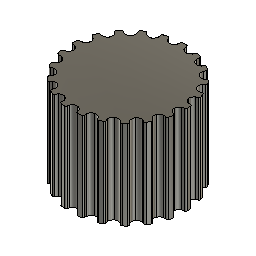
gear_21z (Autodesk Fusion 360 design; units mm, degrees)
Autodesk Fusion 360 part; units mm, degrees
sketch "Sketch1" plane through (0, 0, 0) normal (0, 0, 1) x (1, 0, 0) in component "gt2 pulley"
  circle A0 centre (0, 0) radius 6.6845 construction
  circle A1 centre (0, 0) radius 5.6805 construction
  line L0 (0, 0) -> (0, 6.6845) construction
  line L1 (0, 0) -> (0.9963, 6.6098) construction
  line L2 (0, 0) -> (1.4116, 6.5338) construction
  circle A2 centre (0, 0) radius 6.4305 construction
  arc A3 (0.358, 6.2782) -> (0.3948, 6.0167) centre (1.358, 6.2855) ccw
  circle A4 centre (0, 0) radius 6.2805 construction
  arc A5 (0.2129, 6.427) -> (0, 6.4305) centre (0, 0) ccw
  arc A6 (0.358, 6.2782) -> (0.2129, 6.427) centre (0.208, 6.2771) ccw
  arc A7 (0.3948, 6.0167) -> (0.8466, 5.6171) centre (0.9294, 6.1659) ccw
  arc A8 (0, 6.4305) -> (-0.2129, 6.427) centre (0, 0) ccw
  arc A9 (-0.2129, 6.427) -> (-0.358, 6.2782) centre (-0.208, 6.2771) ccw
  arc A10 (-0.3948, 6.0167) -> (-0.358, 6.2782) centre (-1.358, 6.2855) ccw
  arc A11 (-0.8464, 5.6171) -> (-0.3948, 6.0167) centre (-0.9294, 6.1659) ccw
  arc A12 (0.8466, 5.6171) -> (-0.8466, 5.6171) centre (0, 0) ccw
  point P0 (1.358, 6.2855)
  point P1 (0, 6.4305)
  dimension "d18" = 13.369
  dimension "d19" = 8.571
  dimension "d22" = 1.004
  dimension "d24" = 0.75
  dimension "d26" = 1
  dimension "d27" = 0.15
  dimension "d28" = 0.15
  dimension "d47" = 0.555
  dimension "d52" = 3.812
  constraint coincident A0.centre A1.centre
  constraint coincident A0 L0.end
  constraint vertical L0
  constraint coincident A0 L1.end
  constraint coincident A0 L2.end
  constraint concentric A1 A2
  constraint coincident A1 A7.end
  constraint coincident L1 A7.end
  constraint coincident A2 P0
  constraint coincident L2 P0
  constraint coincident P0 A3.centre
  constraint coincident A2 P1
  constraint coincident L0 P1
  constraint concentric A2 A4
  constraint coincident P1 A5.end
  constraint coincident A4 A6.centre
  constraint coincident A3.start A6.start
  constraint tangent A3 A6
  constraint tangent A3 A7
  constraint symmetric L0 A7.end A12.end
  constraint symmetric L0 A3.start A9.end
  constraint symmetric L0 A3.end A10.start
  constraint symmetric L0 A3 A10
  constraint symmetric L0 A5.start A8.end
  constraint symmetric L0 P1 A5.end
  constraint symmetric L0 A5 A8
  constraint symmetric L0 A6 A9
  constraint symmetric L0 A7 A11
  constraint coincident A1 A11.start
  constraint tangent A1 A7
  constraint coincident L1 A7.centre
  measures "d18" diameter of A0
  measures "d19" angle of L0 L1
  measures "d22" distance of A0 A1
  measures "d24" distance of A1 A2
  measures "d26" radius of A3
  measures "d27" distance of A2 A4
  measures "d28" radius of A6
  measures "d47" radius of A7
extrude "Extrude1" add sketch "Sketch1" along normal blind 10 makes body 1
pattern_circular "C-Pattern1" count 21 over 360 about axis through (0, 0, 1.75) along (0, 0, 1) of bodies 1 makes body 2 at (-2.293, 5.1971, 6.6667) makes body 3 at (-3.7231, 4.2903, 6.6667) makes body 4 at (-4.8222, 3.0023, 6.6667) makes body 5 at (-5.0973, 2.5072, 6.6667) makes body 6 at (-5.6756, -0.2358, 6.6667) makes body 7 at (-5.6474, -0.6125, 3.3333) makes body 8 at (-4.5566, -3.392, 6.6667) makes body 9 at (-3.7941, -4.2277, 6.6667) makes body 10 at (-3.0422, -4.7972, 3.3333) makes body 11 at (-0.7533, -5.6303, 6.6667) makes body 12 at (1.4928, -5.4808, 6.6667) makes body 13 at (1.8538, -5.3695, 3.3333) makes body 14 at (3.3542, -4.5845, 3.3333) makes body 15 at (4.5565, -3.3922, 3.3333) makes body 16 at (5.6474, -0.6127, 6.6667) makes body 17 at (5.6756, -0.236, 3.3333) makes body 18 at (5.0112, 2.675, 6.6667) makes body 19 at (4.0001, 4.0333, 6.6667) makes body 20 at (3.7232, 4.2902, 3.3333) makes body 21 at (2.2932, 5.197, 3.3333)
sketch "Sketch2" plane through (0, 0, 10) normal (0, 0, 1) x (-1, 0, 0)
  arc A0 (-3.8324, -4.9856) -> (-3.7964, -5.1903) centre (-3.7079, -5.0692) ccw
  arc A1 (-3.7964, -5.1903) -> (-3.4445, -5.4302) centre (0, 0) ccw
  arc A2 (-3.4445, -5.4302) -> (-3.2408, -5.3889) centre (-3.3641, -5.3035) ccw
  arc A3 (-3.0631, -5.1936) -> (-3.2408, -5.3889) centre (-2.4187, -5.9583) ccw
  arc A4 (-2.4649, -5.1179) -> (-3.0631, -5.1936) centre (-2.7055, -5.618) ccw
  arc A5 (-3.8637, -4.1641) -> (-2.4649, -5.1179) centre (0, 0) ccw
  arc A6 (-3.7155, -4.7488) -> (-3.8637, -4.1641) centre (-4.2412, -4.571) ccw
  arc A7 (-3.8324, -4.9856) -> (-3.7155, -4.7488) centre (-4.6628, -4.4283) ccw
  circle A8 centre (0, 0) radius 5.6805
  constraint concentric A1 A8
extrude "Extrude2" add sketch "Sketch2" against normal blind 10 contours A5 A8 bodies 1 2 3 4 5 6 7 8 9 10 11 12 13 14 15 16 17 18 19 20 21
extrude "Extrude4" [suppressed] in component "gt2 pulley"
pattern_circular "C-Pattern7" [suppressed] in component "gt2 pulley"
extrude "Extrude3" [suppressed] in component "gt2 pulley"
pattern_circular "C-Pattern6" [suppressed] in component "gt2 pulley"
extrude "Extrude2'" [suppressed] in component "gt2 pulley"
pattern_circular "C-Pattern5" [suppressed] in component "gt2 pulley"
extrude "Extrude1'" [suppressed] in component "gt2 pulley"
pattern_circular "C-Pattern4" [suppressed] in component "gt2 pulley"
pattern_circular "C-Pattern3" [suppressed] in component "gt2 pulley"
pattern_circular "C-Pattern2" [suppressed] in component "gt2 pulley"
pattern_circular "C-Pattern1'" [suppressed] in component "gt2 pulley"
copy_body "Body->Comp1" [suppressed] in component "Component"
copy_body "Body->Comp2" [suppressed] in component "Component'"
copy_body "Body->Comp3" [suppressed] in component "Component''"
copy_body "Body->Comp4" [suppressed] in component "Component'''"
copy_body "Body->Comp5" [suppressed] in component "Component''''"
copy_body "Body->Comp6" [suppressed] in component "Component'''''"
copy_body "Body->Comp7" [suppressed] in component "Component''''''"
copy_body "Body->Comp8" [suppressed] in component "Component'''''''"
copy_body "Body->Comp9" [suppressed] in component "Component''''''''"
copy_body "Body->Comp10" [suppressed] in component "Component'''''''''"
copy_body "Body->Comp11" [suppressed] in component "Component''''''''''"
copy_body "Body->Comp12" [suppressed] in component "Component'''''''''''"
copy_body "Body->Comp13" [suppressed] in component "Component''''''''''''"
copy_body "Body->Comp14" [suppressed] in component "Component'''''''''''''"
copy_body "Body->Comp15" [suppressed] in component "Component''''''''''''''"
copy_body "Body->Comp16" [suppressed] in component "Component'''''''''''''''"
copy_body "Body->Comp17" [suppressed] in component "Component''''''''''''''''"
copy_body "Body->Comp18" [suppressed] in component "Component'''''''''''''''''"
copy_body "Body->Comp19" [suppressed] in component "Component''''''''''''''''''"
copy_body "Body->Comp20" [suppressed] in component "Component'''''''''''''''''''"
component "gt2 pulley" placed x (1, 0, 0) y (0, 1, 0) z (0, 0, 1) at (0, 0, 0)
equation "NumTeeth = 21" comment "min 20"
equation "ToothPitch = 2 mm"
equation "PullyDia = NumTeeth * ToothPitch / PI"
equation "ToothAng = ( ( 360 / NumTeeth ) * 1 deg )"
equation "TransOffsetAngle = ToothAng * 0.2"
equation "Sholulder_Radius = 0.15 mm"
equation "Root_Radius = 0.555 mm"
equation "TransRadius = 1 mm"
equation "ToolHeight = 0.75 mm"
equation "PLD = 0.254 mm"
equation "d18 = PullyDia"
equation "d19 = ToothAng / 2"
equation "d22 = PLD + ToolHeight"
equation "d24 = ToolHeight"
equation "d26 = TransRadius"
equation "d27 = Sholulder_Radius"
equation "d31 = NumTeeth"
equation "d33 = NumTeeth"
equation "d35 = NumTeeth"
equation "d37 = NumTeeth"
equation "d41 = NumTeeth"
equation "d45 = NumTeeth"
equation "d47 = Root_Radius"
equation "d50 = NumTeeth"
